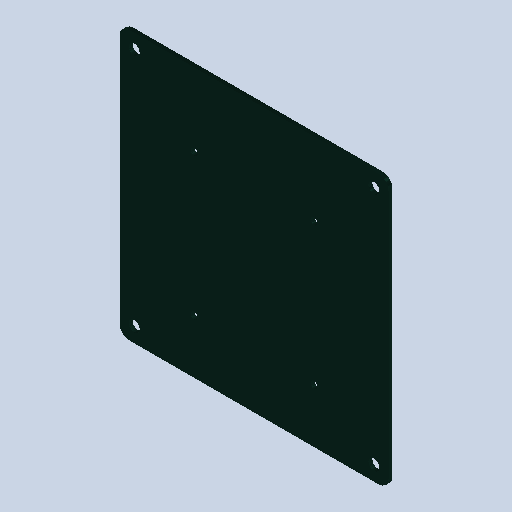
# Autodesk Inventor part: pcb
Saved by Autodesk Inventor 2024 (Build 280153000, 153)
## iProperties
Part Number: pcb
Material: Generic
Document SubType Name: Modeling
Designer: Thomas
Appearance: PCB
pcb_fixation_ecart: 98.000 mm
pcb_size: 110.000 mm
Author: Thomas
Autodesk Inventor part; units mm, degrees
ref_plane "YZ Plane" through (0, 0, 0) normal (1, 0, 0) x (0, 1, 0)
ref_plane "XZ Plane" through (0, 0, 0) normal (0, 1, 0) x (-1, 0, 0)
ref_plane "XY Plane" through (0, 0, 0) normal (0, 0, 1) x (1, 0, 0)
sketch "Sketch1" plane through (0, 0, 0) normal (0, 0, 1) x (1, 0, 0)
  line L0 (0, 0) -> (-110, 0)
  line L1 (-110, 0) -> (-110, 110)
  line L2 (-110, 110) -> (0, 110)
  line L3 (0, 110) -> (0, 0)
  dimension "pcb_size" = 110
  dimension "d1" = 110
  constraints: 8 end point, 2 parallel, 1 horizontal, 1 perpendicular
  measures "pcb_size" distance of L2.end L0.start
  measures "d1" distance of L0.start L0.end
extrude "Extrusion1" add sketch "Sketch1" along normal blind 1.6
fillet "Fillet1" radius 4 4 edges at (0, 0, 0.8) (0, 110, 0.8) (-110, 110, 0.8) (-110, 0, 0.8)
sketch "Sketch2" plane through (0, 0, 1.6) normal (0, 0, 1) x (1, 0, 0)
  line L0 (0, 4) -> (0, 106) projected
  line L1 (-4, 110) -> (-106, 110) projected
  line L2 (-55, 110) -> (-55, 0) construction
  line L3 (-106, 0) -> (-4, 0) construction
  line L4 (0, 55) -> (-110, 55) construction
  line L5 (-110, 106) -> (-110, 4) construction
  point P0 (0, 0)
  point P1 (-6, 104)
  point P2 (-104, 104)
  point P3 (-6, 6)
  point P4 (-104, 6)
  dimension "d12" = 6
  dimension "d13" = 6
  dimension "pcb_fixation_ecart" = 98
  dimension "d28" = 98
  constraints: 4 end point, 4 midpoint, 3 symmetric about line
  measures "d12" distance from line of L0 point (-6, 104)
  measures "d13" distance from line of L1 point (-6, 104)
  measures "pcb_fixation_ecart" distance of point (-6, 104) point (-104, 104)
  measures "d28" distance of point (-104, 6) point (-104, 104)
hole "Hole1" at (-6, 104, 1.6) at (-6, 6, 1.6) at (-104, 6, 1.6) at (-104, 104, 1.6) direction (0, 0, -1) diameter 4.5 end through all clearance for "Countersunk Flat Head Screw DIN EN ISO 2009" size "M4" standard "DIN"
sketch "Sketch3" plane through (-55, 69.5861, 1.6) normal (0, 0, 1) x (1, 0, 0)
  line L0 (-24.5, -47.5861) -> (24.5, -47.5861) construction
  line L1 (-24.5, -47.5861) -> (-24.5, 10.4139) construction
  line L2 (0, -47.5861) -> (0, 10.4139) construction
  line L3 (-24.5, 10.4139) -> (24.5, 10.4139) construction
  line L4 (24.5, 10.4139) -> (24.5, -47.5861) construction
  line L5 (0, -4) -> (-24.5, -47.5861) construction
  line L6 (55, -65.5861) -> (55, 36.4139) projected
  line L7 (-55, 36.4139) -> (-55, -65.5861) projected
  line L8 (51, 40.4139) -> (-51, 40.4139) projected
  dimension "d16" = 58
  dimension "d15" = 49
  dimension "d17" = 50
  dimension "d24" = 110
  dimension "d25" = 55
  dimension "d26" = 30
  constraints: 12 end point, 2 horizontal, 2 horizontal alignment, 2 midpoint, 2 vertical, 2 vertical alignment, 1 perpendicular, 1 point on line
  measures "d16" distance of L1.end L0.start
  measures "d15" distance of L0.start L0.end
  measures "d17" distance of L5.start L0.start
  measures "d24" distance between parallel lines of L6 L7
  measures "d25" distance between parallel lines of L2 L7
  measures "d26" distance between parallel lines of L8 L3
hole "Hole2" at (-79.5, 22, 1.6) at (-79.5, 80, 1.6) at (-30.5, 22, 1.6) at (-30.5, 80, 1.6) direction (0, 0, -1) diameter 2.9 end through all
equation "\"d13\" = d12"
equation "\"d25\" = 0.5 * d24"
body "Solid1"
